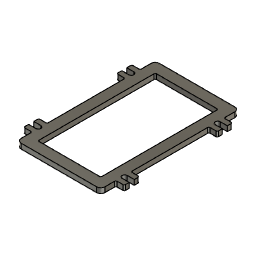
Hopper Flange v2 (Autodesk Fusion 360 design; units mm, degrees)
Autodesk Fusion 360 part; units mm, degrees
sketch "Sketch1" plane through (0, 0, 0) normal (0, 0, 1) x (1, 0, 0)
  line L0 (0, 0) -> (-90, 0)
  line L1 (0, 25) -> (-72, 25)
  line L2 (-75, 28) -> (-75, 165)
  arc A0 (-75, 28) -> (-72, 25) centre (-72, 28) ccw
  arc A1 (-100, 10) -> (-90, 0) centre (-90, 10) ccw
  line L3 (-103, 72) -> (-117, 72)
  line L4 (-120, 69) -> (-120, 39)
  line L5 (-117, 36) -> (-103, 36)
  line L6 (-120, 54) -> (-100, 54) construction
  line L7 (-103, 60) -> (-120, 60)
  line L8 (-120, 60) -> (-120, 48)
  line L9 (-120, 48) -> (-103, 48)
  arc A2 (-103, 48) -> (-103, 60) centre (-103, 54) ccw
  line L10 (-100, 10) -> (-100, 33)
  line L11 (-100, 75) -> (-100, 165)
  arc A3 (-117, 72) -> (-120, 69) centre (-117, 69) ccw
  arc A4 (-120, 39) -> (-117, 36) centre (-117, 39) ccw
  arc A5 (-103, 72) -> (-100, 75) centre (-103, 75) ccw
  arc A6 (-100, 33) -> (-103, 36) centre (-103, 33) ccw
  line L12 (0, 180) -> (0, -75.868) construction
  line L13 (75, 28) -> (75, 165)
  line L14 (103, 72) -> (117, 72)
  line L15 (0, 0) -> (90, 0)
  line L16 (103, 60) -> (120, 60)
  line L17 (120, 60) -> (120, 48)
  line L18 (100, 75) -> (100, 165)
  arc A7 (117, 36) -> (120, 39) centre (117, 39) ccw
  arc A8 (90, 0) -> (100, 10) centre (90, 10) ccw
  line L19 (100, 10) -> (100, 33)
  line L20 (120, 69) -> (120, 39)
  arc A9 (103, 60) -> (103, 48) centre (103, 54) ccw
  arc A10 (120, 69) -> (117, 72) centre (117, 69) ccw
  arc A11 (72, 25) -> (75, 28) centre (72, 28) ccw
  arc A12 (103, 36) -> (100, 33) centre (103, 33) ccw
  line L21 (120, 48) -> (103, 48)
  line L22 (0, 25) -> (72, 25)
  arc A13 (100, 75) -> (103, 72) centre (103, 75) ccw
  line L23 (120, 54) -> (100, 54) construction
  line L24 (117, 36) -> (103, 36)
  line L25 (100, 165) -> (-100, 165) construction
  line L26 (0, 150) -> (0, 405.868) construction
  line L27 (75, 302) -> (75, 165)
  line L28 (103, 258) -> (117, 258)
  line L29 (0, 305) -> (-72, 305)
  line L30 (-103, 270) -> (-120, 270)
  line L31 (120, 276) -> (100, 276) construction
  line L32 (-75, 302) -> (-75, 165)
  line L33 (0, 330) -> (90, 330)
  arc A14 (-103, 270) -> (-103, 282) centre (-103, 276) ccw
  line L34 (-103, 258) -> (-117, 258)
  arc A15 (-103, 294) -> (-100, 297) centre (-103, 297) ccw
  arc A16 (75, 302) -> (72, 305) centre (72, 302) ccw
  line L35 (-100, 320) -> (-100, 297)
  line L36 (-117, 294) -> (-103, 294)
  line L37 (-120, 261) -> (-120, 291)
  arc A17 (100, 320) -> (90, 330) centre (90, 320) ccw
  arc A18 (-72, 305) -> (-75, 302) centre (-72, 302) ccw
  line L38 (117, 294) -> (103, 294)
  arc A19 (117, 258) -> (120, 261) centre (117, 261) ccw
  arc A20 (-120, 261) -> (-117, 258) centre (-117, 261) ccw
  line L39 (120, 270) -> (120, 282)
  arc A21 (103, 282) -> (103, 270) centre (103, 276) ccw
  arc A22 (-90, 330) -> (-100, 320) centre (-90, 320) ccw
  arc A23 (-100, 255) -> (-103, 258) centre (-103, 255) ccw
  line L40 (-120, 270) -> (-120, 282)
  line L41 (120, 282) -> (103, 282)
  arc A24 (120, 291) -> (117, 294) centre (117, 291) ccw
  arc A25 (-117, 294) -> (-120, 291) centre (-117, 291) ccw
  line L42 (-120, 276) -> (-100, 276) construction
  arc A26 (100, 297) -> (103, 294) centre (103, 297) ccw
  line L43 (0, 330) -> (-90, 330)
  line L44 (-120, 282) -> (-103, 282)
  line L45 (100, 320) -> (100, 297)
  arc A27 (103, 258) -> (100, 255) centre (103, 255) ccw
  line L46 (103, 270) -> (120, 270)
  line L47 (120, 261) -> (120, 291)
  line L48 (-100, 255) -> (-100, 165)
  line L49 (100, 255) -> (100, 165)
  line L50 (0, 305) -> (72, 305)
  point P0 (-100, 0)
  point P1 (-75, 25)
  point P2 (-120, 72)
  point P3 (-120, 36)
  point P4 (120, 36)
  point P5 (120, 72)
  point P6 (100, 0)
  point P7 (75, 25)
  point P8 (-75, 305)
  point P9 (0, 330)
  point P10 (120, 258)
  point P11 (120, 294)
  point P12 (75, 305)
  point P13 (-100, 330)
  point P14 (-120, 294)
  point P15 (-120, 258)
  point P16 (100, 330)
  dimension "d16" = 100
  dimension "d17" = 165
  dimension "d18" = 25
  dimension "d19" = 25
  dimension "d20" = 140
  dimension "d21" = 3
  dimension "d22" = 10
  dimension "d23" = 12
  dimension "d24" = 3
  dimension "d25" = 36
  dimension "d28" = 3
  dimension "d29" = 3
  dimension "d30" = 3
  dimension "d31" = 54
  dimension "d32" = 36
  constraint coincident L0.start L15.start
  constraint horizontal L0
  constraint perpendicular L0 L10
  constraint horizontal L1
  constraint perpendicular L1 L2
  constraint coincident P1 L1
  constraint coincident P1 L2
  constraint tangent L1 A0
  constraint tangent L2 A0
  constraint coincident P0 L0
  constraint coincident P0 L10
  constraint tangent L0 A1
  constraint tangent A1 L10
  constraint horizontal L3
  constraint vertical L4
  constraint horizontal L5
  constraint coincident A2.centre L6
  constraint horizontal L7
  constraint vertical L8
  constraint horizontal L9
  constraint coincident L4 L8.end
  constraint tangent L7 A2
  constraint tangent L9 A2
  constraint collinear L10 L11
  constraint coincident L4 L6.start
  constraint coincident P2 L3
  constraint coincident P2 L4
  constraint tangent L3 A3
  constraint tangent L4 A3
  constraint coincident P3 L4
  constraint coincident P3 L5
  constraint tangent L4 A4
  constraint tangent L5 A4
  constraint equal A3 A4
  constraint tangent L11 A5
  constraint tangent L3 A5
  constraint tangent L10 A6
  constraint tangent L5 A6
  constraint vertical L12
  constraint symmetric L0.start L12 L15.start
  constraint symmetric P0 L12 P6
  constraint symmetric L11.end L12 L18.end
  constraint symmetric L1.start L12 L22.start
  constraint symmetric P1 L12 P7
  constraint symmetric L2.end L12 L13.end
  constraint symmetric L1.end L12 A11.start
  constraint symmetric L2.start L12 L13.start
  constraint symmetric A0 L12 A11
  constraint symmetric L0.end L12 L15.end
  constraint symmetric A1.start L12 A8.end
  constraint symmetric A1 L12 A8
  constraint symmetric P2 L12 P5
  constraint symmetric P3 L12 P4
  constraint symmetric L6.start L12 L23.start
  constraint symmetric L6.end L12 L23.end
  constraint symmetric L7.start L12 L16.start
  constraint symmetric L7.end L12 L16.end
  constraint symmetric L8.end L12 L17.end
  constraint symmetric L9.end L12 A9.end
  constraint symmetric A2 L12 A9
  constraint symmetric L3.end L12 L14.end
  constraint symmetric L4.start L12 L20.start
  constraint symmetric A3 L12 A10
  constraint symmetric L4.end L12 A7.end
  constraint symmetric L5.start L12 A7.start
  constraint symmetric A4 L12 A7
  constraint symmetric L11.start L12 L18.start
  constraint symmetric L3.start L12 L14.start
  constraint symmetric A5 L12 A13
  constraint symmetric L10.end L12 L19.end
  constraint symmetric L5.end L12 A12.start
  constraint symmetric A6 L12 A12
  constraint symmetric L0.start L25 P9
  constraint symmetric P0 L25 P13
  constraint symmetric L11.end L25 L48.end
  constraint symmetric L1.start L25 L29.start
  constraint symmetric P1 L25 P8
  constraint symmetric L2.end L25 L32.end
  constraint symmetric L1.end L25 L29.end
  constraint symmetric L2.start L25 L32.start
  constraint symmetric A0 L25 A18
  constraint symmetric L0.end L25 A22.start
  constraint symmetric A1.start L25 L35.start
  constraint symmetric A1 L25 A22
  constraint symmetric P2 L25 P15
  constraint symmetric P3 L25 P14
  constraint symmetric L6.start L25 L42.start
  constraint symmetric L6.end L25 L42.end
  constraint symmetric L7.start L25 L30.start
  constraint symmetric L7.end L25 L30.end
  constraint symmetric L8.end L25 L40.end
  constraint symmetric L9.end L25 A14.end
  constraint symmetric A2 L25 A14
  constraint symmetric L3.end L25 L34.end
  constraint symmetric L4.start L25 L37.start
  constraint symmetric A3 L25 A20
  constraint symmetric L4.end L25 L37.end
  constraint symmetric L5.start L25 L36.start
  constraint symmetric A4 L25 A25
  constraint symmetric L11.start L25 A23.start
  constraint symmetric L3.start L25 L34.start
  constraint symmetric A5 L25 A23
  constraint symmetric L10.end L25 A15.end
  constraint symmetric L5.end L25 A15.start
  constraint symmetric A6 L25 A15
  constraint symmetric L12.start L25 L26.start
  constraint symmetric L12.end L25 L26.end
  constraint symmetric A12.start L25 L38.end
  constraint symmetric L16.start L25 A21.end
  constraint symmetric L13.end L25 L27.end
  constraint symmetric L20.start L25 A19.end
  constraint symmetric L14.end L25 L28.end
  constraint symmetric A9.end L25 A21.start
  constraint symmetric L16.end L25 L39.start
  constraint symmetric L17.end L25 L39.end
  constraint symmetric A11.start L25 A16.end
  constraint symmetric P4 L25 P11
  constraint symmetric A7.end L25 A24.start
  constraint symmetric L14.start L25 L28.start
  constraint symmetric L13.start L25 L27.start
  constraint symmetric L18.end L25 L49.end
  constraint symmetric P5 L25 P10
  constraint symmetric L15.end L25 L33.end
  constraint symmetric P6 L25 P16
  constraint symmetric L23.end L25 L31.end
  constraint symmetric L18.start L25 A27.end
  constraint symmetric A8.end L25 A17.start
  constraint symmetric P7 L25 P12
  constraint symmetric A7.start L25 L38.start
  constraint symmetric L23.start L25 L31.start
  constraint symmetric L19.end L25 A26.start
  constraint symmetric A7 L25 A24
  constraint symmetric A8 L25 A17
  constraint symmetric A9 L25 A21
  constraint symmetric A10 L25 A19
  constraint symmetric A11 L25 A16
  constraint symmetric A12 L25 A26
  constraint symmetric A13 L25 A27
  measures "d16" distance of L0.start P0
  measures "d17" distance of P0 L11.end
  measures "d18" distance of L0 L1
  measures "d19" distance of L2 L10
  measures "d20" distance of P1 L2.end
  measures "d21" radius of A0
  measures "d22" radius of A1
  measures "d23" diameter of A2
  measures "d24" distance of A2 L10
  measures "d25" distance of P2 P3
  measures "d28" radius of A3
  measures "d29" radius of A5
  measures "d30" radius of A6
  measures "d31" distance of L0 A2.centre
  measures "d32" distance of L0 L5
extrude "Extrude1" add sketch "Sketch1" along normal blind 12 contours L0 A1 L3 L4 L5 L7 L9 A2 L10 L11 A3 A4 A5 A6 L14 L15 L16 L18 A7 A8 L19 L20 A9 A10 A12 L21 A13 L24 L28 L30 L33 A14 L34 A15 L35 L36 L37 A17 L38 A19 A20 A21 A22 A23 L41 A24 A25 A26 L43 L44 L45 A27 L46 L47 L48 L49
equation "width = 200 mm"
equation "length = 330 mm"
equation "outer_corner_radius = 10 mm"
equation "inner_corner_radius = 3 mm"
equation "edge_width = 25 mm"
equation "thickness = 12 mm"
equation "notch_diameter = 12 mm"
equation "notch_ear_extension = 20 mm"
equation "notch_ear_width = 12 mm"
equation "notch_inset = 3 mm"
equation "notch_to_edge_distance = 54 mm"
equation "d16 = width / 2"
equation "d17 = length / 2"
equation "d18 = edge_width"
equation "d19 = edge_width"
equation "d20 = ( length / 2 ) - ( edge_width )"
equation "d21 = inner_corner_radius"
equation "d22 = outer_corner_radius"
equation "d23 = notch_diameter"
equation "d24 = notch_inset"
equation "d25 = notch_diameter + ( notch_ear_width * 2 )"
equation "notch_ear_corner_radius = 3 mm"
equation "d28 = notch_ear_corner_radius"
equation "d29 = notch_ear_corner_radius"
equation "d30 = notch_ear_corner_radius"
equation "d31 = notch_to_edge_distance"
equation "d32 = notch_to_edge_distance - ( notch_diameter / 2 ) - notch_ear_width"
equation "d33 = thickness"
